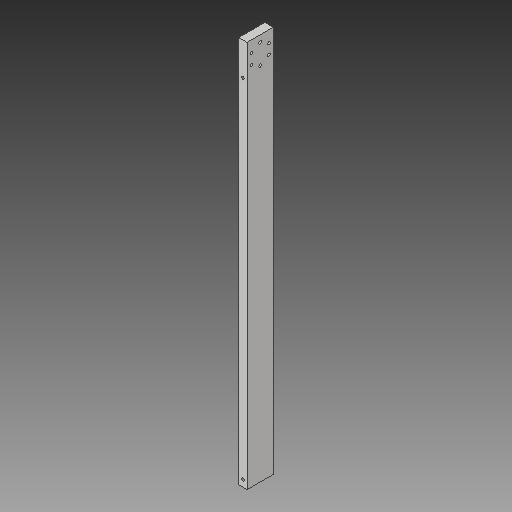
# Autodesk Inventor part: GlyphPlateLeftSide
Saved by Autodesk Inventor 2017 (Build 210142000, 142)
## iProperties
Created: 2018-01-27
Part Number: GlyphPlateLeftSide
Material: Generic
Document SubType Name: Modeling
Designer: User
Density: 1 g/cm^3
Appearance: Default
Author: User
Autodesk Inventor part; units mm, degrees
ref_plane "YZ Plane" through (0, 0, 0) normal (1, 0, 0) x (0, 1, 0)
ref_plane "XZ Plane" through (0, 0, 0) normal (0, 1, 0) x (-1, 0, 0)
ref_plane "XY Plane" through (0, 0, 0) normal (0, 0, 1) x (1, 0, 0)
sketch "Sketch1" plane through (0, 0, 0) normal (0, 0, 1) x (1, 0, 0)
  line L0 (0, 0) -> (8.0518, 0)
  line L1 (8.0518, 0) -> (8.0518, 374.65)
  line L2 (8.0518, 374.65) -> (0, 374.65)
  line L3 (0, 374.65) -> (0, 0)
  dimension "d0" = 8.0518
  dimension "d1" = 374.65
  constraints: 8 end point, 2 parallel, 1 horizontal, 1 perpendicular
  measures "d0" distance of L2.end L1.end
  measures "d1" distance of L1.end L0.end
extrude "Extrusion1" add sketch "Sketch1" along normal blind 25.4
sketch "Sketch2" plane through (0, 0, 25.4) normal (0, 0, 1) x (1, 0, 0)
  line L0 (0, 0) -> (8.0518, 0) projected
  line L1 (4.0259, 0) -> (4.0259, 6.35)
  circle A0 centre (4.0259, 6.35) radius 1.778
  line L2 (8.0518, 374.65) -> (0, 374.65) projected
  line L3 (4.0259, 374.65) -> (4.0259, 342.9)
  circle A1 centre (4.0259, 342.9) radius 1.778
  dimension "d4" = 6.35
  dimension "d5" = 3.556
  dimension "d6" = 31.75
  dimension "d7" = 3.556
  constraints: 4 coincident, 4 end point, 2 centre point, 2 midpoint, 2 vertical
  measures "d4" distance of L1.start L1.end
  measures "d5" diameter of A0
  measures "d6" distance of L3.start L3.end
  measures "d7" diameter of A1
hole "Hole1" at (4.0259, 342.9, 25.4) at (4.0259, 6.35, 25.4) direction (0, 0, -1) diameter 2.6416 depth 25.4 tip angle 118 thread size "6-32 UNC" class "2B" standard "ANSI Unified Screw Threads"
sketch "Sketch3" plane through (8.0518, 0, 0) normal (1, 0, 0) x (0, 0, -1)
  line L0 (0, 374.65) -> (-25.4, 374.65) projected
  circle A0 centre (-12.7, 358.521) radius 9.779
  point P0 (0, 0)
  point P1 (-12.7, 368.3)
  point P2 (-21.1689, 363.4105)
  point P3 (-21.1689, 353.6315)
  point P4 (-12.7, 348.742)
  point P5 (-4.2311, 353.6315)
  point P6 (-4.2311, 363.4105)
  dimension "d22" = 360
  constraints: 1 centre point, 7 other
hole "Hole2" at (8.0518, 368.3, 12.7) at (8.0518, 363.4105, 21.1689) at (8.0518, 353.6315, 21.1689) at (8.0518, 348.742, 12.7) at (8.0518, 353.6315, 4.2311) at (8.0518, 363.4105, 4.2311) direction (-1, 0, 0) diameter 2.7178 depth 25.4 tip angle 118
body "Solid1"
